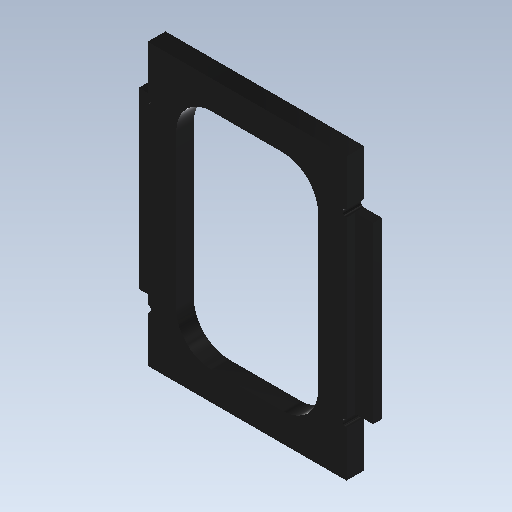
# Autodesk Inventor part: コックピット_2_サブフレーム_1
Saved by Autodesk Inventor 2020 (Build 240168000, 168)
## iProperties
Created: 2016-05-24
Part Number: コックピット_2_サブフレーム_1
Material: アセタール樹脂、黒
Document SubType Name: Modeling
Designer: hiroaki
Density: 1.425 g/cm^3
Appearance: 滑らか - 黒
Mass: 14.5273 g
Surface Area: 66.6596 cm^2
Volume: 10.1946 cm^3
Category: コックピット
Author: hiroaki
Autodesk Inventor part; units mm, degrees
ref_plane "YZ Plane" through (0, 0, 0) normal (1, 0, 0) x (0, 1, 0)
ref_plane "XZ Plane" through (0, 0, 0) normal (0, 1, 0) x (-1, 0, 0)
ref_plane "XY Plane" through (0, 0, 0) normal (0, 0, 1) x (1, 0, 0)
sketch "スケッチ1" plane through (0, 0, 0) normal (0, 0, 1) x (1, 0, 0)
  line L0 (-28, -39.55) -> (28, -39.55) construction
  line L1 (28, -39.55) -> (28, 39.55) construction
  line L2 (28, 39.55) -> (-28, 39.55) construction
  line L3 (-28, 39.55) -> (-28, -39.55) construction
  line L4 (-28, -39.55) -> (28, 39.55) construction
  line L5 (28, -39.55) -> (-28, 39.55) construction
  line L6 (-28, 26.65) -> (-28, 39.55)
  line L7 (-28, 39.55) -> (28, 39.55)
  line L8 (28, 39.55) -> (28, 26.65)
  line L9 (-28, 24.55) -> (-33, 24.55)
  line L10 (-33, 24.55) -> (-33, -24.55)
  line L11 (-33, -24.55) -> (-28, -24.55)
  line L12 (-28, -26.65) -> (-28, -39.55)
  line L13 (-28, -39.55) -> (28, -39.55)
  line L14 (28, -39.55) -> (28, -26.65)
  line L15 (28, 24.55) -> (33, 24.55)
  line L16 (33, 24.55) -> (33, -24.55)
  line L17 (33, -24.55) -> (28, -24.55)
  arc A0 (-28, 24.55) -> (-28, 26.65) centre (-28, 25.6) ccw
  arc A1 (-28, -26.65) -> (-28, -24.55) centre (-28, -25.6) ccw
  arc A2 (28, -24.55) -> (28, -26.65) centre (28, -25.6) ccw
  line L18 (0, 0) -> (0, 39.55) construction
  line L19 (0, 0) -> (28, 0) construction
  arc A3 (28, 26.65) -> (28, 24.55) centre (28, 25.6) ccw
  dimension "d9" = 56
  dimension "d12" = 79.1
  dimension "d13" = 15
  dimension "d39" = 15
  dimension "d40" = 1.05
  dimension "d41" = 5
  constraints: 40 end point, 10 perpendicular, 8 point on circle, 5 symmetric about line, 4 centre point, 4 collinear, 4 midpoint, 4 point on line, 3 horizontal, 2 horizontal alignment, 2 parallel, 2 vertical, 1 equal radius, 1 tangent, 1 other
  measures "d9" distance of L1.end L2.end
  measures "d12" distance of L0.end L1.end
  measures "d13" distance between parallel lines of L9 L2
  measures "d39" distance between parallel lines of L0 L11
  measures "d40" radius of A0
  measures "d41" distance of L9.start L9.end
extrude "押し出し1" add sketch "スケッチ1" along normal blind 5
sketch "スケッチ2" plane through (0, 0, 5) normal (0, 0, 1) x (1, 0, 0)
  line L0 (-28, 39.55) -> (-28, 26.65) projected
  line L1 (28, 39.55) -> (-28, 39.55) projected
  line L2 (-67.7785, 43.014) -> (-28, 43.014)
  line L3 (-28, 43.014) -> (-28, -43.014)
  line L4 (-28, -43.014) -> (-67.7785, -43.014)
  line L5 (-67.7785, -43.014) -> (-67.7785, 43.014)
  line L6 (67.7785, 43.014) -> (28, 43.014)
  line L7 (28, 43.014) -> (28, -43.014)
  line L8 (28, -43.014) -> (67.7785, -43.014)
  line L9 (67.7785, -43.014) -> (67.7785, 43.014)
  line L10 (0, 0) -> (0, 39.55) construction
  line L11 (0, 0) -> (33, 0) construction
  line L12 (33, 24.55) -> (33, -24.55) construction
  constraints: 20 end point, 4 parallel, 2 horizontal, 2 midpoint, 2 perpendicular, 2 symmetric about line, 1 collinear, 3 other
extrude "押し出し2" cut sketch "スケッチ2" against normal blind 2.5
sketch "スケッチ3" plane through (0, 0, 5) normal (0, 0, 1) x (1, 0, 0)
  line L0 (28, 39.55) -> (-28, 39.55) projected
  line L1 (-28, 39.55) -> (-28, 26.65) projected
  line L2 (-20, -31.55) -> (20, -31.55)
  line L3 (20, -31.55) -> (20, 31.55)
  line L4 (20, 31.55) -> (-20, 31.55)
  line L5 (-20, 31.55) -> (-20, -31.55)
  line L6 (-20, -31.55) -> (20, 31.55) construction
  line L7 (20, -31.55) -> (-20, 31.55) construction
  point P0 (0, 0)
  dimension "d47" = 8
  dimension "d48" = 8
  constraints: 12 end point, 2 midpoint, 2 parallel, 1 horizontal, 1 perpendicular
  measures "d47" distance between parallel lines of L1 L5
  measures "d48" distance between parallel lines of L0 L4
extrude "押し出し3" cut sketch "スケッチ3" against normal blind 10
fillet "フィレット1" radius 10 4 edges at (-20, 31.55, 2.5) (20, 31.55, 2.5) (20, -31.55, 2.5) (-20, -31.55, 2.5)
equation "\"d12\" = d18"
equation "\"d13\" = d28"
equation "\"d39\" = d13"
equation "\"d47\" = d48"
equation "\"d18\" = 79.1"
equation "\"d28\" = 15"
